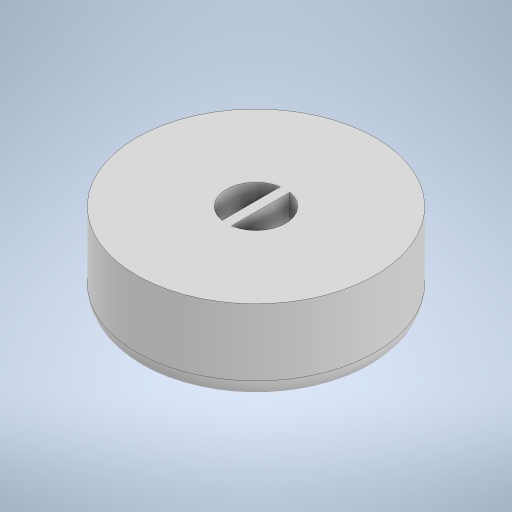
# Autodesk Inventor part: volumeKnob
Saved by Autodesk Inventor 2023 (Build 270158000, 158)
## iProperties
Created: 2022-07-14
Part Number: volumeKnob
Material: Generic
Document SubType Name: Modeling
Designer: Zain Ali
Density: 1 g/cm^3
Appearance: Default
Author: Zain Ali
Autodesk Inventor part; units mm, degrees
ref_plane "YZ Plane" through (0, 0, 0) normal (1, 0, 0) x (0, 1, 0)
ref_plane "XZ Plane" through (0, 0, 0) normal (0, 1, 0) x (-1, 0, 0)
ref_plane "XY Plane" through (0, 0, 0) normal (0, 0, 1) x (1, 0, 0)
sketch "Sketch1" plane through (0, 0, 0) normal (0, 1, 0) x (-1, 0, 0)
  circle A0 centre (0, 0) radius 12.5
  circle A1 centre (0, 0) radius 3.1
  line L0 (-0.5, 3.0594) -> (-0.5, -3.0594)
  line L1 (0.5, -3.0594) -> (0.5, 3.0594)
  line L2 (0.5, 3.0594) -> (-0.5, -3.0594) construction
  line L3 (-0.5, 3.0594) -> (0.5, -3.0594) construction
  dimension "d0" = 6.2
  dimension "d1" = 25
  dimension "d3" = 1
  constraints: 8 end point, 2 coincident, 2 midpoint, 1 centre point, 1 parallel, 1 vertical, 3 other
  measures "d1" diameter of A0
  measures "d3" distance between parallel lines of L0 L1
extrude "Extrusion1" add sketch "Sketch1" along normal blind 7
extrude "Extrusion2" add sketch "Sketch1" along normal blind 7 contours L1 A1 L0
extrude "Extrusion3" add sketch "Sketch1" against normal blind 2 contours A0 | A1 L1 | L1 A1 L0 | L0 A1
fillet "Fillet1" radius 2 1 edges at (12.5, -2, 0)
body "Solid1"
